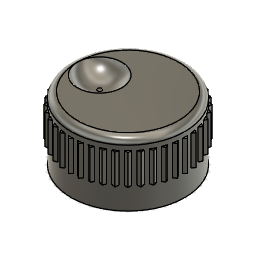
USB_knob_the v4 (Autodesk Fusion 360 design; units mm, degrees)
Autodesk Fusion 360 part; units mm, degrees
sketch "Sketch1" plane through (0, 0, 0) normal (0, 1, 0) x (1, 0, 0)
  circle A0 centre (0, 0) radius 17.95
  circle A1 centre (0, 0) radius 3.05
  line L0 (-3.05, 0) -> (3.05, 0)
  line L1 (-1.5, 0) -> (-1.5, 2.6557)
  line L2 (-1.5, 0) -> (-1.5, -2.6557)
  circle A2 centre (0, 0) radius 3.55
  line L3 (0, 17.95) -> (0, 18.75)
  line L4 (0, 18.75) -> (0.8485, 17.9015)
  line L5 (0, 18.75) -> (1.2, 18.75) construction
  line L6 (0, 18.75) -> (-0.8485, 17.9015)
  line L7 (-2.9331, 18.5192) -> (-1.9623, 17.8138)
  line L8 (-2.9331, 18.5192) -> (-3.6385, 17.5483)
  line L9 (-5.7941, 17.8323) -> (-4.7249, 17.2875)
  line L10 (-5.7941, 17.8323) -> (-6.3389, 16.7631)
  line L11 (-8.5123, 16.7064) -> (-7.3711, 16.3356)
  line L12 (-8.5123, 16.7064) -> (-8.8831, 15.5651)
  line L13 (-11.021, 15.1691) -> (-9.8357, 14.9813)
  line L14 (-11.021, 15.1691) -> (-11.2087, 13.9838)
  line L15 (-13.2583, 13.2583) -> (-12.0583, 13.2583)
  line L16 (-13.2583, 13.2583) -> (-13.2583, 12.0583)
  line L17 (-15.1691, 11.021) -> (-13.9838, 11.2087)
  line L18 (-15.1691, 11.021) -> (-14.9813, 9.8357)
  line L19 (-16.7064, 8.5123) -> (-15.5651, 8.8831)
  line L20 (-16.7064, 8.5123) -> (-16.3356, 7.3711)
  line L21 (-17.8323, 5.7941) -> (-16.7631, 6.3389)
  line L22 (-17.8323, 5.7941) -> (-17.2875, 4.7249)
  line L23 (-18.5192, 2.9331) -> (-17.5483, 3.6385)
  line L24 (-18.5192, 2.9331) -> (-17.8138, 1.9623)
  line L25 (-18.75, 0) -> (-17.9015, 0.8485)
  line L26 (-18.75, 0) -> (-17.9015, -0.8485)
  line L27 (-18.5192, -2.9331) -> (-17.8138, -1.9623)
  line L28 (-18.5192, -2.9331) -> (-17.5483, -3.6385)
  line L29 (-17.8323, -5.7941) -> (-17.2875, -4.7249)
  line L30 (-17.8323, -5.7941) -> (-16.7631, -6.3389)
  line L31 (-16.7064, -8.5123) -> (-16.3356, -7.3711)
  line L32 (-16.7064, -8.5123) -> (-15.5651, -8.8831)
  line L33 (-15.1691, -11.021) -> (-14.9813, -9.8357)
  line L34 (-15.1691, -11.021) -> (-13.9838, -11.2087)
  line L35 (-13.2583, -13.2583) -> (-13.2583, -12.0583)
  line L36 (-13.2583, -13.2583) -> (-12.0583, -13.2583)
  line L37 (-11.021, -15.1691) -> (-11.2087, -13.9838)
  line L38 (-11.021, -15.1691) -> (-9.8357, -14.9813)
  line L39 (-8.5123, -16.7064) -> (-8.8831, -15.5651)
  line L40 (-8.5123, -16.7064) -> (-7.3711, -16.3356)
  line L41 (-5.7941, -17.8323) -> (-6.3389, -16.7631)
  line L42 (-5.7941, -17.8323) -> (-4.7249, -17.2875)
  line L43 (-2.9331, -18.5192) -> (-3.6385, -17.5483)
  line L44 (-2.9331, -18.5192) -> (-1.9623, -17.8138)
  line L45 (0, -18.75) -> (-0.8485, -17.9015)
  line L46 (0, -18.75) -> (0.8485, -17.9015)
  line L47 (2.9331, -18.5192) -> (1.9623, -17.8138)
  line L48 (2.9331, -18.5192) -> (3.6385, -17.5483)
  line L49 (5.7941, -17.8323) -> (4.7249, -17.2875)
  line L50 (5.7941, -17.8323) -> (6.3389, -16.7631)
  line L51 (8.5123, -16.7064) -> (7.3711, -16.3356)
  line L52 (8.5123, -16.7064) -> (8.8831, -15.5651)
  line L53 (11.021, -15.1691) -> (9.8357, -14.9813)
  line L54 (11.021, -15.1691) -> (11.2087, -13.9838)
  line L55 (13.2583, -13.2583) -> (12.0583, -13.2583)
  line L56 (13.2583, -13.2583) -> (13.2583, -12.0583)
  line L57 (15.1691, -11.021) -> (13.9838, -11.2087)
  line L58 (15.1691, -11.021) -> (14.9813, -9.8357)
  line L59 (16.7064, -8.5123) -> (15.5651, -8.8831)
  line L60 (16.7064, -8.5123) -> (16.3356, -7.3711)
  line L61 (17.8323, -5.7941) -> (16.7631, -6.3389)
  line L62 (17.8323, -5.7941) -> (17.2875, -4.7249)
  line L63 (18.5192, -2.9331) -> (17.5483, -3.6385)
  line L64 (18.5192, -2.9331) -> (17.8138, -1.9623)
  line L65 (18.75, 0) -> (17.9015, -0.8485)
  line L66 (18.75, 0) -> (17.9015, 0.8485)
  line L67 (18.5192, 2.9331) -> (17.8138, 1.9623)
  line L68 (18.5192, 2.9331) -> (17.5483, 3.6385)
  line L69 (17.8323, 5.7941) -> (17.2875, 4.7249)
  line L70 (17.8323, 5.7941) -> (16.7631, 6.3389)
  line L71 (16.7064, 8.5123) -> (16.3356, 7.3711)
  line L72 (16.7064, 8.5123) -> (15.5651, 8.8831)
  line L73 (15.1691, 11.021) -> (14.9813, 9.8357)
  line L74 (15.1691, 11.021) -> (13.9838, 11.2087)
  line L75 (13.2583, 13.2583) -> (13.2583, 12.0583)
  line L76 (13.2583, 13.2583) -> (12.0583, 13.2583)
  line L77 (11.021, 15.1691) -> (11.2087, 13.9838)
  line L78 (11.021, 15.1691) -> (9.8357, 14.9813)
  line L79 (8.5123, 16.7064) -> (8.8831, 15.5651)
  line L80 (8.5123, 16.7064) -> (7.3711, 16.3356)
  line L81 (5.7941, 17.8323) -> (6.3389, 16.7631)
  line L82 (5.7941, 17.8323) -> (4.7249, 17.2875)
  line L83 (2.9331, 18.5192) -> (3.6385, 17.5483)
  line L84 (2.9331, 18.5192) -> (1.9623, 17.8138)
  circle A3 centre (0, 0) radius 15.95
  point P0 (-1.5, 0)
  dimension "d1" = 35.9
  dimension "d4" = 6.1
  dimension "d5" = 4.55
  dimension "d12" = 7.1
  dimension "d15" = 0.8
  dimension "d16" = 45
  dimension "d17" = 1.2
  dimension "d19" = 360
  dimension "d25" = -2
  constraint coincident A0.centre A1.centre
  constraint concentric A0 A1
  constraint coincident A1 L0.start
  constraint coincident A1 L0.end
  constraint horizontal L0
  constraint coincident L0 P0
  constraint coincident P0 L1.start
  constraint coincident A1 L1.end
  constraint perpendicular L0 L1
  constraint coincident A1 L2.end
  constraint perpendicular L0 L2
  constraint concentric A0 A2
  constraint coincident A0 L3.start
  constraint vertical L3
  constraint horizontal L5
  constraint symmetric L4.start L3 L5.start
  constraint symmetric L3 L4.end L6.end
  measures "d1" diameter of A0
  measures "d4" diameter of A1
  measures "d5" distance of L0.end P0
  measures "d12" diameter of A2
  measures "d15" distance of L3.start L3.end
  measures "d16" angle of L4 L5
  measures "d17" distance of L3.end L4.end
extrude "Extrude1" add sketch "Sketch1" along normal blind 20 contours A0 | A1 L0 L1 | A1 L0 L2 | A1 L0 L1 | A1 L0 L2 | A2 | A3
extrude "Extrude2" cut sketch "Sketch1" along normal blind 11.25 contours A1 L0 L1 | A1 L0 L2 | A1 L0 L1 | A1 L0 L2 | A2
extrude "Extrude3" cut sketch "Sketch1" along normal blind 18.6 contours A1 L0 L1 | A1 L0 L2 picked at (1.5221, 0.1508) picked at (1.5221, -0.1508)
chamfer "Chamfer2" distance 12.4 distance2 11.25 1 edges at (-3.3098, 0, 1.2837) measured on face at (13.07, 0, 1.0681)
extrude "Extrude4" add sketch "Sketch1" 1 faces at (17.1563, 0, 1.6841) along normal blind 20 contours A0 L65 L66 | A0 L67 L68 | A0 L63 L64 | A0 L69 L70 | A0 L61 L62 | A0 L71 L72 | A0 L59 L60 | A0 L73 L74 | A0 L57 L58 | A0 L75 L76 | A0 L55 L56 | A0 L77 L78 | A0 L53 L54 | A0 L79 L80 | A0 L51 L52 | A0 L81 L82 | A0 L49 L50 | A0 L83 L84 | A0 L47 L48 | A0 L3 L4 | A0 L45 L46 | A0 L3 L6 | A0 L43 L44 | A0 L7 L8 | A0 L41 L42 | A0 L9 L10 | A0 L39 L40 | A0 L11 L12 | A0 L37 L38 | A0 L13 L14 | A0 L35 L36 | A0 L15 L16 | A0 L33 L34 | A0 L17 L18 | A0 L31 L32 | A0 L19 L20 | A0 L29 L30 | A0 L21 L22 | A0 L27 L28 | A0 L23 L24 | A0 L25 L26
extrude "Extrude5" add sketch "Sketch1" against normal blind 10 contours A0
sketch "Sketch3" plane through (0, -10, 0) normal (0, -1, 0) x (1, 0, 0)
  circle A0 centre (0, 0) radius 15.95
  circle A1 centre (0, 0) radius 17.95
  circle A2 centre (0, 0) radius 20
  dimension "d28" = 40
  constraint coincident A0.centre A1.centre
  measures "d28" diameter of A2
extrude "Extrude6" cut sketch "Sketch3" against normal blind 10 contours A1
extrude "Extrude7" cut sketch "Sketch3" against normal blind 17 contours A2
sketch "Sketch4" plane through (0, 20, 0) normal (0, 1, 0) x (-1, 0, 0)
  arc A0 (17.9313, 0.8187) -> (17.8386, 1.9965) centre (0, 0) ccw
  line L0 (17.8386, 1.9965) -> (18.5192, 2.9331)
  line L1 (18.5192, 2.9331) -> (17.5825, 3.6137)
  arc A1 (17.5825, 3.6137) -> (17.3067, 4.7625) centre (0, 0) ccw
  line L2 (17.3067, 4.7625) -> (17.8323, 5.7941)
  line L3 (17.8323, 5.7941) -> (16.8007, 6.3197)
  arc A2 (16.8007, 6.3197) -> (16.3486, 7.4112) centre (0, 0) ccw
  line L4 (16.3486, 7.4112) -> (16.7064, 8.5123)
  line L5 (16.7064, 8.5123) -> (15.6053, 8.8701)
  arc A3 (15.6053, 8.8701) -> (14.988, 9.8774) centre (0, 0) ccw
  line L6 (14.988, 9.8774) -> (15.1691, 11.021)
  line L7 (15.1691, 11.021) -> (14.0255, 11.2021)
  arc A4 (14.0255, 11.2021) -> (13.2583, 12.1005) centre (0, 0) ccw
  line L8 (13.2583, 12.1005) -> (13.2583, 13.2583)
  line L9 (13.2583, 13.2583) -> (12.1005, 13.2583)
  arc A5 (12.1005, 13.2583) -> (11.2021, 14.0255) centre (0, 0) ccw
  line L10 (11.2021, 14.0255) -> (11.021, 15.1691)
  line L11 (11.021, 15.1691) -> (9.8774, 14.988)
  arc A6 (9.8774, 14.988) -> (8.8701, 15.6053) centre (0, 0) ccw
  line L12 (8.8701, 15.6053) -> (8.5123, 16.7064)
  line L13 (8.5123, 16.7064) -> (7.4112, 16.3486)
  arc A7 (7.4112, 16.3486) -> (6.3197, 16.8007) centre (0, 0) ccw
  line L14 (6.3197, 16.8007) -> (5.7941, 17.8323)
  line L15 (5.7941, 17.8323) -> (4.7625, 17.3067)
  arc A8 (4.7625, 17.3067) -> (3.6137, 17.5825) centre (0, 0) ccw
  line L16 (3.6137, 17.5825) -> (2.9331, 18.5192)
  line L17 (2.9331, 18.5192) -> (1.9965, 17.8386)
  arc A9 (1.9965, 17.8386) -> (0.8187, 17.9313) centre (0, 0) ccw
  line L18 (0.8187, 17.9313) -> (0, 18.75)
  line L19 (0, 18.75) -> (-0.8187, 17.9313)
  arc A10 (-0.8187, 17.9313) -> (-1.9965, 17.8386) centre (0, 0) ccw
  line L20 (-1.9965, 17.8386) -> (-2.9331, 18.5192)
  line L21 (-2.9331, 18.5192) -> (-3.6137, 17.5825)
  arc A11 (-3.6137, 17.5825) -> (-4.7625, 17.3067) centre (0, 0) ccw
  line L22 (-4.7625, 17.3067) -> (-5.7941, 17.8323)
  line L23 (-5.7941, 17.8323) -> (-6.3197, 16.8007)
  arc A12 (-6.3197, 16.8007) -> (-7.4112, 16.3486) centre (0, 0) ccw
  line L24 (-7.4112, 16.3486) -> (-8.5123, 16.7064)
  line L25 (-8.5123, 16.7064) -> (-8.8701, 15.6053)
  arc A13 (-8.8701, 15.6053) -> (-9.8774, 14.988) centre (0, 0) ccw
  line L26 (-9.8774, 14.988) -> (-11.021, 15.1691)
  line L27 (-11.021, 15.1691) -> (-11.2021, 14.0255)
  arc A14 (-11.2021, 14.0255) -> (-12.1005, 13.2583) centre (0, 0) ccw
  line L28 (-12.1005, 13.2583) -> (-13.2583, 13.2583)
  line L29 (-13.2583, 13.2583) -> (-13.2583, 12.1005)
  arc A15 (-13.2583, 12.1005) -> (-14.0255, 11.2021) centre (0, 0) ccw
  line L30 (-14.0255, 11.2021) -> (-15.1691, 11.021)
  line L31 (-15.1691, 11.021) -> (-14.988, 9.8774)
  arc A16 (-14.988, 9.8774) -> (-15.6053, 8.8701) centre (0, 0) ccw
  line L32 (-15.6053, 8.8701) -> (-16.7064, 8.5123)
  line L33 (-16.7064, 8.5123) -> (-16.3486, 7.4112)
  arc A17 (-16.3486, 7.4112) -> (-16.8007, 6.3197) centre (0, 0) ccw
  line L34 (-16.8007, 6.3197) -> (-17.8323, 5.7941)
  line L35 (-17.8323, 5.7941) -> (-17.3067, 4.7625)
  arc A18 (-17.3067, 4.7625) -> (-17.5825, 3.6137) centre (0, 0) ccw
  line L36 (-17.5825, 3.6137) -> (-18.5192, 2.9331)
  line L37 (-18.5192, 2.9331) -> (-17.8386, 1.9965)
  arc A19 (-17.8386, 1.9965) -> (-17.9313, 0.8187) centre (0, 0) ccw
  line L38 (-17.9313, 0.8187) -> (-18.75, 0)
  line L39 (-18.75, 0) -> (-17.9313, -0.8187)
  arc A20 (-17.9313, -0.8187) -> (-17.8386, -1.9965) centre (0, 0) ccw
  line L40 (-17.8386, -1.9965) -> (-18.5192, -2.9331)
  line L41 (-18.5192, -2.9331) -> (-17.5825, -3.6137)
  arc A21 (-17.5825, -3.6137) -> (-17.3067, -4.7625) centre (0, 0) ccw
  line L42 (-17.3067, -4.7625) -> (-17.8323, -5.7941)
  line L43 (-17.8323, -5.7941) -> (-16.8007, -6.3197)
  arc A22 (-16.8007, -6.3197) -> (-16.3486, -7.4112) centre (0, 0) ccw
  line L44 (-16.3486, -7.4112) -> (-16.7064, -8.5123)
  line L45 (-16.7064, -8.5123) -> (-15.6053, -8.8701)
  arc A23 (-15.6053, -8.8701) -> (-14.988, -9.8774) centre (0, 0) ccw
  line L46 (-14.988, -9.8774) -> (-15.1691, -11.021)
  line L47 (-15.1691, -11.021) -> (-14.0255, -11.2021)
  arc A24 (-14.0255, -11.2021) -> (-13.2583, -12.1005) centre (0, 0) ccw
  line L48 (-13.2583, -12.1005) -> (-13.2583, -13.2583)
  line L49 (-13.2583, -13.2583) -> (-12.1005, -13.2583)
  arc A25 (-12.1005, -13.2583) -> (-11.2021, -14.0255) centre (0, 0) ccw
  line L50 (-11.2021, -14.0255) -> (-11.021, -15.1691)
  line L51 (-11.021, -15.1691) -> (-9.8774, -14.988)
  arc A26 (-9.8774, -14.988) -> (-8.8701, -15.6053) centre (0, 0) ccw
  line L52 (-8.8701, -15.6053) -> (-8.5123, -16.7064)
  line L53 (-8.5123, -16.7064) -> (-7.4112, -16.3486)
  arc A27 (-7.4112, -16.3486) -> (-6.3197, -16.8007) centre (0, 0) ccw
  line L54 (-6.3197, -16.8007) -> (-5.7941, -17.8323)
  line L55 (-5.7941, -17.8323) -> (-4.7625, -17.3067)
  arc A28 (-4.7625, -17.3067) -> (-3.6137, -17.5825) centre (0, 0) ccw
  line L56 (-3.6137, -17.5825) -> (-2.9331, -18.5192)
  line L57 (-2.9331, -18.5192) -> (-1.9965, -17.8386)
  arc A29 (-1.9965, -17.8386) -> (-0.8187, -17.9313) centre (0, 0) ccw
  line L58 (-0.8187, -17.9313) -> (0, -18.75)
  line L59 (0, -18.75) -> (0.8187, -17.9313)
  arc A30 (0.8187, -17.9313) -> (1.9965, -17.8386) centre (0, 0) ccw
  line L60 (1.9965, -17.8386) -> (2.9331, -18.5192)
  line L61 (2.9331, -18.5192) -> (3.6137, -17.5825)
  arc A31 (3.6137, -17.5825) -> (4.7625, -17.3067) centre (0, 0) ccw
  line L62 (4.7625, -17.3067) -> (5.7941, -17.8323)
  line L63 (5.7941, -17.8323) -> (6.3197, -16.8007)
  arc A32 (6.3197, -16.8007) -> (7.4112, -16.3486) centre (0, 0) ccw
  line L64 (7.4112, -16.3486) -> (8.5123, -16.7064)
  line L65 (8.5123, -16.7064) -> (8.8701, -15.6053)
  arc A33 (8.8701, -15.6053) -> (9.8774, -14.988) centre (0, 0) ccw
  line L66 (9.8774, -14.988) -> (11.021, -15.1691)
  line L67 (11.021, -15.1691) -> (11.2021, -14.0255)
  arc A34 (11.2021, -14.0255) -> (12.1005, -13.2583) centre (0, 0) ccw
  line L68 (12.1005, -13.2583) -> (13.2583, -13.2583)
  line L69 (13.2583, -13.2583) -> (13.2583, -12.1005)
  arc A35 (13.2583, -12.1005) -> (14.0255, -11.2021) centre (0, 0) ccw
  line L70 (14.0255, -11.2021) -> (15.1691, -11.021)
  line L71 (15.1691, -11.021) -> (14.988, -9.8774)
  arc A36 (14.988, -9.8774) -> (15.6053, -8.8701) centre (0, 0) ccw
  line L72 (15.6053, -8.8701) -> (16.7064, -8.5123)
  line L73 (16.7064, -8.5123) -> (16.3486, -7.4112)
  arc A37 (16.3486, -7.4112) -> (16.8007, -6.3197) centre (0, 0) ccw
  line L74 (16.8007, -6.3197) -> (17.8323, -5.7941)
  line L75 (17.8323, -5.7941) -> (17.3067, -4.7625)
  arc A38 (17.3067, -4.7625) -> (17.5825, -3.6137) centre (0, 0) ccw
  line L76 (17.5825, -3.6137) -> (18.5192, -2.9331)
  line L77 (18.5192, -2.9331) -> (17.8386, -1.9965)
  arc A39 (17.8386, -1.9965) -> (17.9313, -0.8187) centre (0, 0) ccw
  line L78 (17.9313, -0.8187) -> (18.75, 0)
  line L79 (18.75, 0) -> (17.9313, 0.8187)
  circle A40 centre (0, 0) radius 17.95
  circle A41 centre (0, 0) radius 15.95
  circle A42 centre (8.95, 0.0036) radius 7
  dimension "d33" = 35.9
  dimension "d34" = -2
  dimension "d54" = 14
  constraint concentric A0 A40
  measures "d33" diameter of A40
  measures "d54" diameter of A42
ref_plane "WorkPlane1" through (0, 30, 0) normal (0, 1, 0) x (-1, 0, 0)
sketch "Sketch6" plane through (0, 30, 0) normal (0, 1, 0) x (1, 0, 0)
  circle A0 centre (0, 0) radius 20
  circle A1 centre (0, 0) radius 17.95
  dimension "d45" = 40
  dimension "d46" = 35.9
  constraint coincident A0.centre A1.centre
  measures "d45" diameter of A0
  measures "d46" diameter of A1
extrude "Extrude11" cut sketch "Sketch6" against normal blind 13.5
fillet "Fillet2" radius 2 1 edges at (-16.7353, 20, 6.491)
extrude "Extrude13" cut sketch "Sketch4" against normal blind 4 contours A42
fillet "Fillet3" radius 7 1 edges at (-2.4237, 16, 2.5349)
